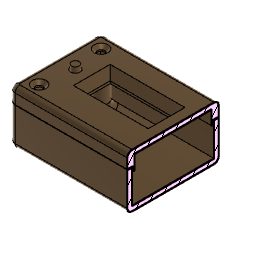
ZPM v1 (Autodesk Fusion 360 design; units mm, degrees)
Autodesk Fusion 360 part; units mm, degrees
sketch "Sketch1" plane through (0, 0, 0) normal (0, 0, 1) x (1, 0, 0)
  line L0 (28.5, -17) -> (-28.5, -17) construction
  line L1 (-28.5, -17) -> (-28.5, 17) construction
  line L2 (-28.5, 17) -> (28.5, 17) construction
  line L3 (28.5, 17) -> (28.5, -17) construction
  line L4 (28.5, -17) -> (-28.5, 17) construction
  line L5 (-28.5, -17) -> (28.5, 17) construction
  line L6 (28.7, -17.2) -> (-28.7, -17.2)
  line L7 (-28.7, -17.2) -> (-28.7, 17.2)
  line L8 (-28.7, 17.2) -> (28.7, 17.2)
  line L9 (28.7, 17.2) -> (28.7, -17.2)
  line L10 (28.7, -17.2) -> (-28.7, 17.2) construction
  line L11 (-28.7, -17.2) -> (28.7, 17.2) construction
  line L12 (30.7, 19.2) -> (30.7, -19.2)
  line L13 (30.7, -19.2) -> (-30.7, -19.2)
  line L14 (-30.7, -19.2) -> (-30.7, 19.2)
  line L15 (-30.7, 19.2) -> (30.7, 19.2)
  circle A0 centre (-24.3, 13) radius 3
  line L16 (0, 2.5) -> (0, 20)
  circle A1 centre (24.3, 13) radius 3
  line L17 (20, 0) -> (2.5, 0)
  circle A2 centre (24.3, -13) radius 3
  circle A3 centre (-24.3, -13) radius 3
  point P0 (-24.3, 13)
  dimension "d1" = 57
  dimension "d2" = 34
  dimension "d3" = 57.4
  dimension "d4" = 34.4
  dimension "d5" = -2
  dimension "d6" = 4
  dimension "d7" = 4.2
  dimension "d8" = 6
  constraint horizontal L0
  constraint perpendicular L0 L1
  constraint parallel L0 L2
  constraint parallel L1 L3
  constraint coincident L4 origin
  constraint coincident L5 origin
  constraint horizontal L6
  constraint perpendicular L6 L7
  constraint parallel L6 L8
  constraint parallel L7 L9
  constraint coincident L10 origin
  constraint coincident L11 origin
  constraint coincident P0 A0.centre
  constraint symmetric A0 L16 A1
  constraint symmetric A0 L17 A3
  constraint symmetric A1 L17 A2
  measures "d1" distance of L1.end L2.end
  measures "d2" distance of L0.end L1.end
  measures "d3" distance of L7.end L8.end
  measures "d4" distance of L6.end L7.end
  measures "d6" distance of L2 P0
  measures "d7" distance of L1 P0
  measures "d8" diameter of A0
extrude "Extrude1" add sketch "Sketch1" along normal blind 14 contours L12 L13 L14 L15 makes body 1
extrude "Extrude2" add sketch "Sketch1" along normal blind 9 separate body contours A0 | A1 | A2 | A3 makes body 2 at (-21.3037, -13.1495, 6) makes body 3 at (27.2963, 12.8505, 6) makes body 4 at (-21.3037, 12.8505, 6) makes body 5 at (27.2963, -13.1495, 6)
extrude "Extrude3" add sketch "Sketch1" against normal blind 2 contours L6 L7 L8 L9 | L12 L13 L14 L15 | A0 | A1 | A2 | A3 bodies 1 2 3 4 5
fillet "Fillet1" radius 2.5 4 edges at (30.7, -19.2, 6) (-30.7, -19.2, 6) (30.7, 19.2, 6) (-30.7, 19.2, 6) on bodies 1
fillet "Fillet2" radius 2 4 edges at (21.503, 11.9152, 0) (21.503, -14.0848, 0) (-27.097, -14.0848, 0) (-27.097, 11.9152, 0) on bodies 1
sketch "Sketch2" plane through (28.7, 0, 0) normal (-1, 0, 0) x (0, -1, 0)
  spline S0 degree 3 poles (10.6251, 0) (10.8542, 0) (11.129, 0.0109) (11.8709, 0.0507) (12.4861, 0.0921) (13, 0.0921) (13.5139, 0.0921) (14.1291, 0.0507) (14.871, 0.0109) (15.1458, 0) (15.3749, 0) knots -0.222895 -0.222895 -0.222895 -0.222895 -0.15416 -0.15416 0 0 0 0.15416 0.15416 0.222895 0.222895 0.222895 0.222895
  line L0 (15.3749, 0) -> (17.2, 0)
  line L1 (17.2, 0) -> (17.2, 14)
  line L2 (17.2, 14) -> (-17.2, 14)
  line L3 (-17.2, 14) -> (-17.2, 0)
  line L4 (-17.2, 0) -> (-15.3749, 0)
  spline S1 degree 3 poles (-15.3749, 0) (-15.1458, 0) (-14.871, 0.0109) (-14.1291, 0.0507) (-13.5139, 0.0921) (-13, 0.0921) (-12.4861, 0.0921) (-11.8709, 0.0507) (-11.129, 0.0109) (-10.8542, 0) (-10.6251, 0) knots -0.222895 -0.222895 -0.222895 -0.222895 -0.15416 -0.15416 0 0 0 0.15416 0.15416 0.222895 0.222895 0.222895 0.222895
  line L5 (-10.6251, 0) -> (10.6251, 0)
  line L6 (-10.6251, 0) -> (10.6251, 0)
  line L7 (-17.2, 0) -> (-17.2, 14)
  line L8 (0, 0) -> (0, 3) construction
  line L9 (5, 0) -> (-5, 0) construction
  line L10 (-5, 0) -> (-5, 6)
  line L11 (-5, 6) -> (5, 6)
  line L12 (5, 6) -> (5, 0)
  line L13 (5, 0) -> (-5, 6) construction
  line L14 (-5, 0) -> (5, 6) construction
  point P0 (0, 3)
  dimension "d19" = 3
  dimension "d20" = 10
  dimension "d21" = 6
  constraint coincident L8.start origin
  constraint perpendicular L5 L8
  constraint horizontal L9
  constraint perpendicular L9 L10
  constraint parallel L9 L11
  constraint parallel L10 L12
  constraint coincident L13 P0
  constraint coincident L14 P0
  constraint coincident P0 L8.end
  measures "d19" distance of L8.start P0
  measures "d20" distance of L10.end L11.end
  measures "d21" distance of L9.end L10.end
extrude "Extrude4" cut sketch "Sketch2" against normal blind 14 contours L5 L6 L10 L11 L12 bodies 1
sketch "Sketch3" plane through (0, 0, 9) normal (0, 0, 1) x (-1, 0, 0)
  circle A0 centre (24.3, -13) radius 3
  circle A1 centre (24.3, -13) radius 1.1
  line L0 (0, -2.5) -> (0, -20)
  circle A2 centre (-24.3, -13) radius 1.1
  line L1 (-20, 0) -> (-2.5, 0)
  circle A3 centre (-24.3, 13) radius 1.1
  circle A4 centre (24.3, 13) radius 1.1
  dimension "d24" = 2.2
  constraint concentric A0 A1
  constraint symmetric A1 L0 A2
  constraint symmetric A1 L1 A4
  constraint symmetric A2 L1 A3
  measures "d24" diameter of A1
extrude "Extrude5" cut sketch "Sketch3" against normal blind 9 contours A1 | A2 | A3 | A4 bodies 1
ref_plane "WorkPlane1" through (-24.3, -13, 16.4) normal (0, 0, 1) x (1, 0, 0)
sketch "Sketch4" plane through (0, 0, 16.4) normal (0, 0, 1) x (1, 0, 0)
  arc A0 (-28.2, 19.2) -> (-30.7, 16.7) centre (-28.2, 16.7) ccw
  line L0 (-30.7, 16.7) -> (-30.7, -16.7)
  arc A1 (-30.7, -16.7) -> (-28.2, -19.2) centre (-28.2, -16.7) ccw
  line L1 (-28.2, -19.2) -> (28.2, -19.2)
  arc A2 (28.2, -19.2) -> (30.7, -16.7) centre (28.2, -16.7) ccw
  line L2 (30.7, -16.7) -> (30.7, 16.7)
  arc A3 (30.7, 16.7) -> (28.2, 19.2) centre (28.2, 16.7) ccw
  line L3 (28.2, 19.2) -> (-28.2, 19.2)
  line L4 (-28.7, 17.2) -> (28.7, 17.2)
  line L5 (28.7, 17.2) -> (28.7, -17.2)
  line L6 (28.7, -17.2) -> (-28.7, -17.2)
  line L7 (-28.7, -17.2) -> (-28.7, 17.2)
  circle A4 centre (-24.3, 13) radius 1.1
  circle A5 centre (-24.3, 13) radius 3
  circle A6 centre (-24.3, -13) radius 1.1
  circle A7 centre (-24.3, -13) radius 3
  circle A8 centre (24.3, -13) radius 1.1
  circle A9 centre (24.3, 13) radius 1.1
  circle A10 centre (24.3, 13) radius 3
  line L8 (28.3, -16.8) -> (-28.3, -16.8)
  line L9 (-28.3, -16.8) -> (-28.3, 16.8)
  line L10 (-28.3, 16.8) -> (28.3, 16.8)
  line L11 (28.3, 16.8) -> (28.3, -16.8)
  line L12 (27.7, 16.2) -> (27.7, -16.2)
  line L13 (27.7, -16.2) -> (-27.7, -16.2)
  line L14 (-27.7, -16.2) -> (-27.7, 16.2)
  line L15 (-27.7, 16.2) -> (27.7, 16.2)
  line L16 (-28.7, 6.2) -> (28.7, 6.2) construction
  line L17 (-28.7, -3.2) -> (28.7, -3.2) construction
  line L18 (-13.7, -17.2) -> (-13.7, 17.2) construction
  line L19 (11.7, -17.2) -> (11.7, 17.2) construction
  line L20 (-13.7, 6.2) -> (11.7, 6.2)
  line L21 (11.7, 6.2) -> (11.7, -3.2)
  line L22 (11.7, -3.2) -> (-13.7, -3.2)
  line L23 (-13.7, -3.2) -> (-13.7, 6.2)
  line L24 (-15.7, -5.2) -> (-15.7, 8.2)
  line L25 (-15.7, 8.2) -> (13.7, 8.2)
  line L26 (13.7, 8.2) -> (13.7, -5.2)
  line L27 (13.7, -5.2) -> (-15.7, -5.2)
  line L28 (-25.3, -17.2) -> (-25.3, 17.2) construction
  line L29 (-28.7, -3) -> (28.7, -3) construction
  line L30 (-28.7, 3.2) -> (28.7, 3.2) construction
  line L31 (26.5, -17.2) -> (26.5, 17.2) construction
  line L32 (-25.3, 3.2) -> (-19.1, 3.2) construction
  line L33 (-19.1, 3.2) -> (-19.1, -3) construction
  line L34 (-19.1, -3) -> (-25.3, -3) construction
  line L35 (-25.3, -3) -> (-25.3, 3.2) construction
  line L36 (-19.1, -3) -> (-25.3, 3.2) construction
  line L37 (26.5, 3.2) -> (20.3, 3.2) construction
  line L38 (20.3, 3.2) -> (20.3, -3) construction
  line L39 (20.3, -3) -> (26.5, -3) construction
  line L40 (26.5, -3) -> (26.5, 3.2) construction
  line L41 (20.3, 3.2) -> (26.5, -3) construction
  circle A11 centre (-22.2, 0.1) radius 3.1
  circle A12 centre (-22.2, 0.1) radius 2
  circle A13 centre (-22.2, 0.1) radius 1.6
  circle A14 centre (23.4, 0.1) radius 3.1
  circle A15 centre (23.4, 0.1) radius 2
  circle A16 centre (23.4, 0.1) radius 1.6
  point P0 (-13.7, 6.2)
  point P1 (11.7, -3.2)
  dimension "d28" = 0.4
  dimension "d29" = 1
  dimension "d30" = 11
  dimension "d31" = 14
  dimension "d32" = 15
  dimension "d33" = 17
  dimension "d34" = -2
  dimension "d39" = 3.4
  dimension "d40" = 14.2
  dimension "d41" = 14
  dimension "d45" = 2.2
  dimension "d46" = 6.2
  dimension "d47" = 6.2
  dimension "d48" = 6.2
  dimension "d49" = 4
  dimension "d50" = 3.2
  dimension "d51" = 6.2
  dimension "d52" = 4
  dimension "d53" = 3.2
  constraint coincident L7 L16.start
  constraint coincident L5 L16.end
  constraint perpendicular L5 L16
  constraint coincident L7 L17.start
  constraint coincident L5 L17.end
  constraint perpendicular L5 L17
  constraint coincident L6 L18.start
  constraint coincident L4 L18.end
  constraint perpendicular L4 L18
  constraint coincident L6 L19.start
  constraint coincident L4 L19.end
  constraint perpendicular L4 L19
  constraint coincident L16 P0
  constraint coincident L18 P0
  constraint coincident L17 P1
  constraint coincident L19 P1
  constraint horizontal L20
  constraint vertical L21
  constraint horizontal L22
  constraint vertical L23
  constraint coincident P1 L21.end
  constraint coincident P0 L20.start
  constraint coincident L6 L28.start
  constraint coincident L4 L28.end
  constraint perpendicular L4 L28
  constraint coincident L7 L29.start
  constraint coincident L5 L29.end
  constraint perpendicular L5 L29
  constraint coincident L7 L30.start
  constraint coincident L5 L30.end
  constraint perpendicular L5 L30
  constraint coincident L6 L31.start
  constraint coincident L4 L31.end
  constraint perpendicular L4 L31
  constraint horizontal L32
  constraint vertical L33
  constraint horizontal L34
  constraint vertical L35
  constraint coincident L30 L32.start
  constraint coincident L28 L32.start
  constraint horizontal L37
  constraint vertical L38
  constraint horizontal L39
  constraint vertical L40
  constraint coincident L31 L37.start
  constraint coincident L30 L37.start
  constraint midpoint L36 A11.centre
  constraint tangent L33 A11
  constraint concentric A11 A12
  constraint concentric A12 A13
  constraint midpoint L41 A14.centre
  constraint concentric A14 A15
  constraint concentric A14 A16
  measures "d30" distance of L4 L16
  measures "d31" distance of L6 L17
  measures "d32" distance of L7 L18
  measures "d33" distance of L5 L19
  measures "d39" distance of L7 L28
  measures "d40" distance of L6 L29
  measures "d41" distance of L4 L30
  measures "d45" distance of L5 L31
  measures "d46" distance of L32.start L32.end
  measures "d47" distance of L37.start L37.end
  measures "d48" distance of L37.start L39.end
  measures "d49" diameter of A12
  measures "d50" diameter of A13
  measures "d51" diameter of A14
  measures "d52" diameter of A15
  measures "d53" diameter of A16
extrude "Extrude6" add sketch "Sketch4" against normal up to surface (2.2 mm away) separate body contours A0 L0 A1 L1 A2 L2 A3 L3 | L4 L5 L6 L7 makes body 6
extrude "Extrude7" add sketch "Sketch4" against normal blind 4 contours L8 L9 L10 L11 bodies 6
extrude "Extrude8" add sketch "Sketch4" along normal blind 2 separate body contours A0 L0 A1 L1 A2 L2 A3 L3 | L4 L5 L6 L7 | L8 L9 L10 L11 | L24 L25 L26 L27 | A11 | A12 | A13 | A14 | A15 | A16 makes body 7 at (-19.1154, -0.2087, 17.0667) makes body 8 at (3.2333, -4.5333, 16.4) makes body 9 at (26.4846, -0.2087, 17.0667) makes body 10 at (9.2333, -18.2, 16.4)
extrude "Extrude9" add sketch "Sketch4" along normal blind 2 from surface at 2 contours A0 L0 A1 L1 A2 L2 A3 L3 | L4 L5 L6 L7 | A4 | A5 | A6 | A7 | A8 | A9 | A10 | L8 L9 L10 L11 | L12 L13 L14 L15 | L24 L25 L26 L27 | A11 | A12 | A13 | A14 | A15 | A16 bodies 8 10
combine "Combine1" operation add target body 8 tool bodies 6
extrude "Extrude10" cut sketch "Sketch4" along normal blind 43 contours A12 | A13 | A15 | A16 bodies 8
extrude "Extrude11" add sketch "Sketch4" along normal blind 6 contours A13 | A16 bodies 9 7
sketch "Sketch5" plane through (0, 0, 20.4) normal (0, 0, 1) x (-1, 0, 0)
  circle A0 centre (-23.4, -0.1) radius 2
  circle A1 centre (22.2, -0.1) radius 2
  line L0 (-11.7, 3.2) -> (13.7, 3.2)
  line L1 (13.7, 3.2) -> (13.7, -6.2)
  line L2 (13.7, -6.2) -> (-11.7, -6.2)
  line L3 (-11.7, -6.2) -> (-11.7, 3.2)
  line L4 (-28.2, -19.2) -> (28.2, -19.2)
  arc A2 (28.2, -19.2) -> (30.7, -16.7) centre (28.2, -16.7) ccw
  line L5 (30.7, -16.7) -> (30.7, 16.7)
  arc A3 (30.7, 16.7) -> (28.2, 19.2) centre (28.2, 16.7) ccw
  line L6 (28.2, 19.2) -> (-28.2, 19.2)
  arc A4 (-28.2, 19.2) -> (-30.7, 16.7) centre (-28.2, 16.7) ccw
  line L7 (-30.7, 16.7) -> (-30.7, -16.7)
  arc A5 (-30.7, -16.7) -> (-28.2, -19.2) centre (-28.2, -16.7) ccw
  point P0 (24.3, -13)
  point P1 (-24.3, -13)
  point P2 (-24.3, 13)
  point P3 (24.3, 13)
hole "Hole1" at (-24.3, 13, 20.4) at (24.3, 13, 20.4) at (24.3, -13, 20.4) at (-24.3, -13, 20.4) direction (0, 0, -1) diameter 3 depth 4 tip angle 118 countersink diameter 5.8 countersink angle 90 bodies 8
chamfer "Chamfer1" distance 3 angle 45 4 edges at (-1, 6.2, 20.4) (11.7, 1.5, 20.4) (-1, -3.2, 20.4) (-13.7, 1.5, 20.4) on bodies 8
fillet "Fillet3" radius 0.4 2 edges at (-23.6917, 0.6786, 18.4) (21.9083, 0.6786, 18.4) on bodies 7 9
fillet "Fillet4" radius 0.6 4 edges at (29.7, 5, 6) (29.7, -5, 6) (29.7, -5, 0) (29.7, 5, 0) on bodies 1
fillet "Fillet5" radius 2 16 edges at (-29.9678, -18.4678, -2) (-30.7, 0, -2) (-29.9678, 18.4678, -2) (0, 19.2, -2) (29.9678, 18.4678, -2) (30.7, 0, -2) (29.9678, -18.4678, -2) (0, -19.2, -2) (-30.7, 0, 20.4) (-29.9678, -18.4678, 20.4) (0, -19.2, 20.4) (29.9678, -18.4678, 20.4) (30.7, 0, 20.4) (29.9678, 18.4678, 20.4) (0, 19.2, 20.4) (-29.9678, 18.4678, 20.4) on bodies 1 8
named bodies: "ZPM_Bottom", "Btn_2", "ZPM_Top", "Btn_1"
